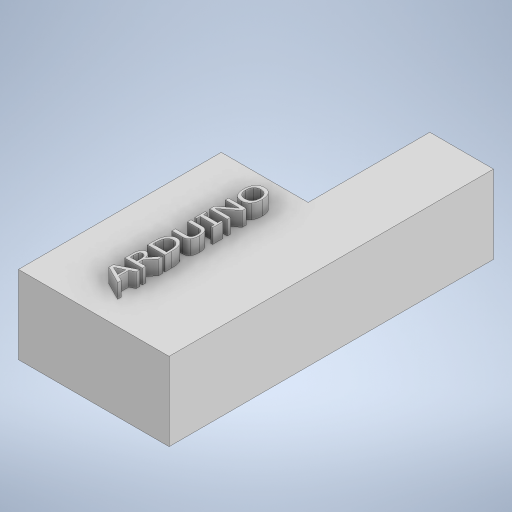
# Autodesk Inventor part: arduino
Saved by Autodesk Inventor 2023 (Build 270158000, 158)
## iProperties
Created: 2022-11-21
Part Number: arduino
Material: Genérico
Document SubType Name: Modeling
Designer: inigo
Density: 1 g/cm^3
Appearance: Valor por defecto
Author: inigo
Autodesk Inventor part; units mm, degrees
ref_plane "YZ Plane" through (0, 0, 0) normal (1, 0, 0) x (0, 1, 0)
ref_plane "XZ Plane" through (0, 0, 0) normal (0, 1, 0) x (-1, 0, 0)
ref_plane "XY Plane" through (0, 0, 0) normal (0, 0, 1) x (1, 0, 0)
sketch "Boceto1" plane through (0, 0, 0) normal (0, 1, 0) x (-1, 0, 0)
  line L0 (26, 35) -> (-26, 35)
  line L1 (-26, 35) -> (-26, -35)
  line L2 (-26, -35) -> (26, -35)
  line L3 (26, -35) -> (26, 35)
  line L4 (26, 35) -> (-26, -35) construction
  line L5 (-26, 35) -> (26, -35) construction
  line L6 (-26, -35) -> (-4, -35)
  line L7 (-4, -35) -> (-4, -77)
  line L8 (-4, -77) -> (-26, -77)
  line L9 (-26, -77) -> (-26, -35)
  point P0 (0, 0)
  dimension "d0" = 52
  dimension "d1" = 70
  dimension "d2" = 22
  dimension "d3" = 42
  constraints: 20 end point, 4 parallel, 2 horizontal, 2 midpoint, 2 perpendicular
  measures "d0" distance of L2.end L1.end
  measures "d1" distance of L1.end L0.end
  measures "d2" distance of L7.end L8.end
  measures "d3" distance of L6.end L7.end
extrude "Extrusión1" add sketch "Boceto1" along normal blind 27
sketch "Boceto2" plane through (0, 27, 0) normal (0, 1, 0) x (1, 0, 0)
  line L0 (-6.1882, -26.7393) -> (-6.1882, -3.0559) construction
  line L1 (-6.1882, -3.0559) -> (46.2207, -3.0559) construction
  line L2 (46.2207, -3.0559) -> (46.2207, -26.7393) construction
  line L3 (46.2207, -26.7393) -> (-6.1882, -26.7393) construction
  line L4 (0.0403, -26.7986) -> (-6.0597, -23.714)
  line L5 (-6.0597, -23.714) -> (-6.0597, -22.2162)
  line L6 (-6.0597, -22.2162) -> (0.0403, -19.1316)
  line L7 (0.0403, -19.1316) -> (0.0403, -20.4168)
  line L8 (0.0403, -20.4168) -> (-1.6651, -21.2473)
  line L9 (-1.6651, -21.2473) -> (-1.6651, -24.7372)
  line L10 (-1.6651, -24.7372) -> (0.0403, -25.5677)
  line L11 (0.0403, -25.5677) -> (0.0403, -26.7986)
  line L12 (-2.3572, -21.5834) -> (-5.2292, -22.9972)
  line L13 (-5.2292, -22.9972) -> (-2.3572, -24.4011)
  line L14 (-2.3572, -24.4011) -> (-2.3572, -21.5834)
  line L15 (0.0403, -11.1828) -> (0.0403, -12.7597)
  line L16 (0.0403, -12.7597) -> (-2.3869, -15.6614)
  line L17 (-2.3869, -15.6614) -> (-2.3869, -17.0505)
  line L18 (-2.3869, -17.0505) -> (0.0403, -17.0505)
  line L19 (0.0403, -17.0505) -> (0.0403, -18.2665)
  line L20 (0.0403, -18.2665) -> (-6.0597, -18.2665)
  line L21 (-6.0597, -18.2665) -> (-6.0597, -15.9086)
  spline S0 degree 2 poles (-6.0597, -15.9086) (-6.0597, -15.1226) (-5.946, -14.0598) (-5.7384, -13.5803) knots 0 0 0 1 2 2 2
  spline S1 degree 2 poles (-5.7384, -13.5803) (-5.5308, -13.1008) (-4.8832, -12.5422) (-4.4037, -12.5422) knots 0 0 0 1 2 2 2
  spline S2 degree 2 poles (-4.4037, -12.5422) (-3.7364, -12.5422) (-2.8317, -13.5605) (-2.6142, -14.4404) knots 0 0 0 1 2 2 2
  line L22 (-2.6142, -14.4404) -> (0.0403, -11.1828)
  spline S3 degree 2 poles (-4.3394, -13.8077) (-4.6064, -13.8077) (-5.0167, -14.0894) (-5.1501, -14.386) knots 0 0 0 1 2 2 2
  spline S4 degree 2 poles (-5.1501, -14.386) (-5.2638, -14.6431) (-5.3578, -15.3351) (-5.3578, -15.8443) knots 0 0 0 1 2 2 2
  line L23 (-5.3578, -15.8443) -> (-5.3578, -17.0505)
  line L24 (-5.3578, -17.0505) -> (-3.0641, -17.0505)
  line L25 (-3.0641, -17.0505) -> (-3.0641, -15.9778)
  spline S5 degree 2 poles (-3.0641, -15.9778) (-3.0641, -15.4587) (-3.1877, -14.6184) (-3.3805, -14.3267) knots 0 0 0 1 2 2 2
  spline S6 degree 2 poles (-3.3805, -14.3267) (-3.5485, -14.0598) (-4.0231, -13.8077) (-4.3394, -13.8077) knots 0 0 0 1 2 2 2
  spline S7 degree 2 poles (-3.0048, -3.2439) (-2.1693, -3.2439) (-0.8248, -4.2573) (-0.4491, -5.1124) knots 0 0 0 1 2 2 2
  spline S8 degree 2 poles (-0.4491, -5.1124) (-0.1574, -5.8045) (0.0403, -7.2381) (0.0403, -8.3503) knots 0 0 0 1 2 2 2
  line L26 (0.0403, -8.3503) -> (0.0403, -10.4561)
  line L27 (0.0403, -10.4561) -> (-6.0597, -10.4561)
  line L28 (-6.0597, -10.4561) -> (-6.0597, -8.375)
  spline S9 degree 2 poles (-6.0597, -8.375) (-6.0597, -7.0848) (-5.8027, -5.6167) (-5.5753, -5.0976) knots 0 0 0 1 2 2 2
  spline S10 degree 2 poles (-5.5753, -5.0976) (-5.1847, -4.2128) (-3.8946, -3.2439) (-3.0048, -3.2439) knots 0 0 0 1 2 2 2
  spline S11 degree 2 poles (-3.0146, -4.5094) (-3.7166, -4.5094) (-4.7102, -5.2113) (-4.992, -5.8984) knots 0 0 0 1 2 2 2
  spline S12 degree 2 poles (-4.992, -5.8984) (-5.1847, -6.3829) (-5.3578, -7.4902) (-5.3578, -8.3107) knots 0 0 0 1 2 2 2
  line L29 (-5.3578, -8.3107) -> (-5.3578, -9.2401)
  line L30 (-5.3578, -9.2401) -> (-0.6616, -9.2401)
  line L31 (-0.6616, -9.2401) -> (-0.6616, -8.3107)
  spline S13 degree 2 poles (-0.6616, -8.3107) (-0.6616, -7.5) (-0.8347, -6.284) (-1.067, -5.7798) knots 0 0 0 1 2 2 2
  spline S14 degree 2 poles (-1.067, -5.7798) (-1.3537, -5.147) (-2.3028, -4.5094) (-3.0146, -4.5094) knots 0 0 0 1 2 2 2
  spline S15 degree 2 poles (0.1688, 1.2743) (0.1688, 0.4685) (-0.1129, -0.7327) (-0.3947, -1.1578) knots 0 0 0 1 2 2 2
  spline S16 degree 2 poles (-0.3947, -1.1578) (-0.7111, -1.6373) (-1.6009, -2.0328) (-2.2534, -2.0328) knots 0 0 0 1 2 2 2
  line L32 (-2.2534, -2.0328) -> (-6.0597, -2.0328)
  line L33 (-6.0597, -2.0328) -> (-6.0597, -0.8167)
  line L34 (-6.0597, -0.8167) -> (-2.2534, -0.8167)
  spline S17 degree 2 poles (-2.2534, -0.8167) (-1.8283, -0.8167) (-1.2548, -0.6586) (-1.0225, -0.4213) knots 0 0 0 1 2 2 2
  spline S18 degree 2 poles (-1.0225, -0.4213) (-0.7753, -0.1741) (-0.5232, 0.6662) (-0.5232, 1.2743) knots 0 0 0 1 2 2 2
  spline S19 degree 2 poles (-0.5232, 1.2743) (-0.5232, 1.8477) (-0.7753, 2.7375) (-1.0225, 2.9797) knots 0 0 0 1 2 2 2
  spline S20 degree 2 poles (-1.0225, 2.9797) (-1.2548, 3.2071) (-1.8233, 3.3752) (-2.2336, 3.3752) knots 0 0 0 1 2 2 2
  line L35 (-2.2336, 3.3752) -> (-6.0597, 3.3752)
  line L36 (-6.0597, 3.3752) -> (-6.0597, 4.5912)
  line L37 (-6.0597, 4.5912) -> (-2.2534, 4.5912)
  spline S21 degree 2 poles (-2.2534, 4.5912) (-1.6157, 4.5912) (-0.7061, 4.2056) (-0.3947, 3.7162) knots 0 0 0 1 2 2 2
  spline S22 degree 2 poles (-0.3947, 3.7162) (-0.108, 3.2812) (0.1688, 2.1196) (0.1688, 1.2743) knots 0 0 0 1 2 2 2
  line L38 (0.0403, 9.5246) -> (0.0403, 5.9753)
  line L39 (0.0403, 5.9753) -> (-0.5826, 5.9753)
  line L40 (-0.5826, 5.9753) -> (-0.5826, 7.1419)
  line L41 (-0.5826, 7.1419) -> (-5.4369, 7.1419)
  line L42 (-5.4369, 7.1419) -> (-5.4369, 5.9753)
  line L43 (-5.4369, 5.9753) -> (-6.0597, 5.9753)
  line L44 (-6.0597, 5.9753) -> (-6.0597, 9.5246)
  line L45 (-6.0597, 9.5246) -> (-5.4369, 9.5246)
  line L46 (-5.4369, 9.5246) -> (-5.4369, 8.358)
  line L47 (-5.4369, 8.358) -> (-0.5826, 8.358)
  line L48 (-0.5826, 8.358) -> (-0.5826, 9.5246)
  line L49 (-0.5826, 9.5246) -> (0.0403, 9.5246)
  line L50 (0.0403, 17.5673) -> (0.0403, 16.203)
  line L51 (0.0403, 16.203) -> (-5.2193, 12.1643)
  line L52 (-5.2193, 12.1643) -> (0.0403, 12.1643)
  line L53 (0.0403, 12.1643) -> (0.0403, 11.0273)
  line L54 (0.0403, 11.0273) -> (-6.0597, 11.0273)
  line L55 (-6.0597, 11.0273) -> (-6.0597, 12.7525)
  line L56 (-6.0597, 12.7525) -> (-1.2301, 16.4303)
  line L57 (-1.2301, 16.4303) -> (-6.0597, 16.4303)
  line L58 (-6.0597, 16.4303) -> (-6.0597, 17.5673)
  line L59 (-6.0597, 17.5673) -> (0.0403, 17.5673)
  spline S23 degree 2 poles (-5.3627, 25.8967) (-4.9574, 26.4158) (-3.771, 26.9941) (-3.0097, 26.9941) knots 0 0 0 1 2 2 2
  spline S24 degree 2 poles (-3.0097, 26.9941) (-2.2682, 26.9941) (-1.067, 26.4306) (-0.6616, 25.8967) knots 0 0 0 1 2 2 2
  spline S25 degree 2 poles (-0.6616, 25.8967) (-0.2365, 25.3332) (0.1688, 23.8403) (0.1688, 22.9456) knots 0 0 0 1 2 2 2
  spline S26 degree 2 poles (0.1688, 22.9456) (0.1688, 22.0162) (-0.2514, 20.5283) (-0.6616, 19.9944) knots 0 0 0 1 2 2 2
  spline S27 degree 2 poles (-0.6616, 19.9944) (-1.067, 19.4655) (-2.2583, 18.902) (-3.0097, 18.902) knots 0 0 0 1 2 2 2
  spline S28 degree 2 poles (-3.0097, 18.902) (-3.7759, 18.902) (-4.9425, 19.4754) (-5.3627, 20.0043) knots 0 0 0 1 2 2 2
  spline S29 degree 2 poles (-5.3627, 20.0043) (-5.7681, 20.5283) (-6.1882, 22.0212) (-6.1882, 22.9456) knots 0 0 0 1 2 2 2
  spline S30 degree 2 poles (-6.1882, 22.9456) (-6.1882, 23.8799) (-5.7532, 25.3777) (-5.3627, 25.8967) knots 0 0 0 1 2 2 2
  spline S31 degree 2 poles (-3.0097, 25.7286) (-3.6128, 25.7286) (-4.5471, 25.3332) (-4.8535, 24.9773) knots 0 0 0 1 2 2 2
  spline S32 degree 2 poles (-4.8535, 24.9773) (-5.1699, 24.6164) (-5.4863, 23.5882) (-5.4863, 22.9505) knots 0 0 0 1 2 2 2
  spline S33 degree 2 poles (-5.4863, 22.9505) (-5.4863, 22.2881) (-5.1798, 21.2995) (-4.8535, 20.9188) knots 0 0 0 1 2 2 2
  spline S34 degree 2 poles (-4.8535, 20.9188) (-4.5421, 20.553) (-3.6029, 20.1675) (-3.0097, 20.1675) knots 0 0 0 1 2 2 2
  spline S35 degree 2 poles (-3.0097, 20.1675) (-1.8085, 20.1675) (-0.5331, 21.6801) (-0.5331, 22.9505) knots 0 0 0 1 2 2 2
  spline S36 degree 2 poles (-0.5331, 22.9505) (-0.5331, 24.2209) (-1.8085, 25.7286) (-3.0097, 25.7286) knots 0 0 0 1 2 2 2
  point P0 (0, 0)
  constraints: 2 other
extrude "Extrusión2" add sketch "Boceto2" along normal blind 5
